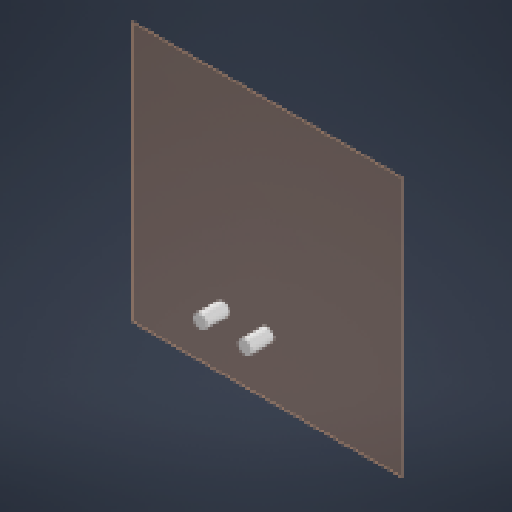
# Autodesk Inventor part: BaseEngranes
Saved by Autodesk Inventor 2026.2 (Build 302298010, 298A)
## iProperties
Created: 2026-04-16
Part Number: BaseEngranes
Material: Genérico
Document SubType Name: Modeling
Designer: Jose Carlos
Density: 1 g/cm^3
Appearance: Valor por defecto
Author: Jose Carlos
Autodesk Inventor part; units mm, degrees
ref_plane "YZ Plane" through (0, 0, 0) normal (1, 0, 0) x (0, 1, 0)
ref_plane "XZ Plane" through (0, 0, 0) normal (0, 1, 0) x (-1, 0, 0)
ref_plane "XY Plane" through (0, 0, 0) normal (0, 0, 1) x (1, 0, 0)
ref_plane "Plano de trabajo1" through (0, 0, 0) normal (0, 0, 1) x (1, 0, 0)
sketch "Boceto1" plane through (0, 0, 0) normal (0, 0, 1) x (1, 0, 0)
  circle A0 centre (-10, -5) radius 1.5 projected
  line L0 (0, 38.6) -> (0, -35.6) construction
  circle A1 centre (10, -5) radius 1.5
  line L1 (27.5, 25) -> (-27.5, 25) construction
  point P0 (0, 0)
  constraints: 2 end point, 1 centre point, 1 symmetric about line, 1 vertical, 3 other
extrude "Extrusión1" add sketch "Boceto1" along normal blind 5
